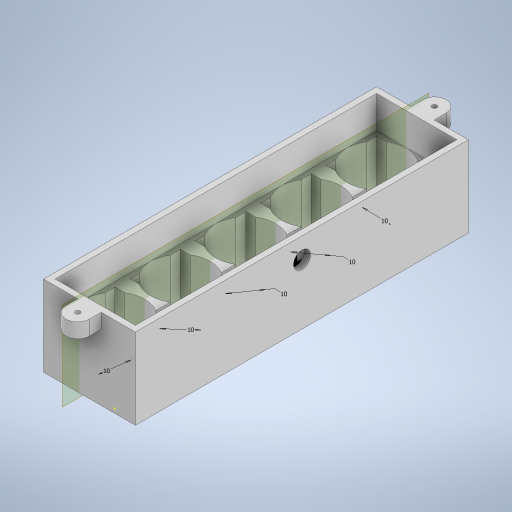
# Autodesk Inventor part: Suporte 4 EletroImã
Saved by Autodesk Inventor 2023 (Build 270158000, 158)
## iProperties
Created: 2023-03-28
Part Number: Suporte 4 EletroImã
Material: Genérico
Document SubType Name: Modeling
Designer: Inteli
Density: 1 g/cm^3
Appearance: Padrão
Author: Inteli
## iProperties of the stored document Suporte 4 EletroImã_3DPrint.ipt
Created: 2023-03-29
Part Number: Suporte 4 EletroImã_3DPrint
Material: Genérico
Document SubType Name: Modeling
Designer: Inteli
Density: 1 g/cm^3
Appearance: Padrão
Author: Inteli
Autodesk Inventor part; units mm, degrees
ref_plane "YZ Plane" through (0, 0, 0) normal (1, 0, 0) x (0, 1, 0)
ref_plane "XZ Plane" through (0, 0, 0) normal (0, 1, 0) x (-1, 0, 0)
ref_plane "XY Plane" through (0, 0, 0) normal (0, 0, 1) x (1, 0, 0)
sketch "Esboço1" plane through (0, 0, 0) normal (0, 1, 0) x (-1, 0, 0)
  circle A0 centre (12.15, -12.15) radius 10.15
  line L0 (0, 0) -> (24.3, 0)
  line L1 (24.3, 0) -> (24.3, -113.5)
  line L2 (24.3, -113.5) -> (0, -113.5)
  line L3 (0, -113.5) -> (0, 0)
  line L4 (20.8, -20.8) -> (3.5, -20.8)
  line L5 (3.5, -20.8) -> (3.5, -3.5)
  line L6 (3.5, -3.5) -> (20.8, -3.5)
  line L7 (20.8, -3.5) -> (20.8, -20.8)
  circle A1 centre (12.15, -34.45) radius 10.15
  line L8 (20.8, -43.1) -> (3.5, -43.1)
  line L9 (3.5, -43.1) -> (3.5, -25.8)
  line L10 (3.5, -25.8) -> (20.8, -25.8)
  line L11 (20.8, -25.8) -> (20.8, -43.1)
  circle A2 centre (12.15, -56.75) radius 10.15
  line L12 (20.8, -65.4) -> (3.5, -65.4)
  line L13 (3.5, -65.4) -> (3.5, -48.1)
  line L14 (3.5, -48.1) -> (20.8, -48.1)
  line L15 (20.8, -48.1) -> (20.8, -65.4)
  circle A3 centre (12.15, -79.05) radius 10.15
  line L16 (20.8, -87.7) -> (3.5, -87.7)
  line L17 (3.5, -87.7) -> (3.5, -70.4)
  line L18 (3.5, -70.4) -> (20.8, -70.4)
  line L19 (20.8, -70.4) -> (20.8, -87.7)
  line L20 (0, -113.5) -> (-7, -113.5)
  line L21 (-7, -113.5) -> (-7, 0)
  line L22 (-7, 0) -> (0, 0)
  line L23 (0, -111.5) -> (-5, -111.5)
  line L24 (-5, -111.5) -> (-5, -2)
  line L25 (-5, -2) -> (0, -2)
  circle A4 centre (12.15, -101.35) radius 10.15
  line L26 (20.8, -110) -> (3.5, -110)
  line L27 (3.5, -110) -> (3.5, -92.7)
  line L28 (3.5, -92.7) -> (20.8, -92.7)
  line L29 (20.8, -92.7) -> (20.8, -110)
  point P0 (20.8, -84.3604)
  point P1 (17.4604, -87.7)
  point P2 (6.8396, -87.7)
  point P3 (3.5, -84.3604)
  point P4 (3.5, -73.7396)
  point P5 (6.8396, -70.4)
  point P6 (17.4604, -70.4)
  point P7 (20.8, -73.7396)
  point P8 (20.8, -62.0604)
  point P9 (17.4604, -65.4)
  point P10 (6.8396, -65.4)
  point P11 (3.5, -62.0604)
  point P12 (3.5, -51.4396)
  point P13 (6.8396, -48.1)
  point P14 (17.4604, -48.1)
  point P15 (20.8, -51.4396)
  point P16 (20.8, -39.7604)
  point P17 (17.4604, -43.1)
  point P18 (6.8396, -43.1)
  point P19 (3.5, -39.7604)
  point P20 (3.5, -29.1396)
  point P21 (6.8396, -25.8)
  point P22 (17.4604, -25.8)
  point P23 (20.8, -29.1396)
  point P24 (20.8, -17.4604)
  point P25 (17.4604, -20.8)
  point P26 (6.8396, -20.8)
  point P27 (3.5, -17.4604)
  point P28 (3.5, -6.8396)
  point P29 (6.8396, -3.5)
  point P30 (17.4604, -3.5)
  point P31 (20.8, -6.8396)
  point P32 (6.8396, -62.0604)
  point P33 (0, -111.5)
  point P34 (6.8396, -110)
  point P35 (3.5, -106.6604)
  point P36 (3.5, -96.0396)
  point P37 (6.8396, -92.7)
  point P38 (17.4604, -92.7)
  point P39 (20.8, -96.0396)
  point P40 (20.8, -106.6604)
  point P41 (17.4604, -110)
  dimension "d0" = 20.3
  dimension "d24" = 22.3
  dimension "d39" = 12.15
  dimension "d41" = 7
  dimension "d42" = 2
  dimension "d96" = 3.5
  dimension "d102" = 5
  constraints: 60 end point, 6 perpendicular, 5 centre point, 5 horizontal, 4 parallel, 1 vertical, 32 other
  measures "d0" diameter of A0
  measures "d24" distance of A0.centre A1.centre
  measures "d39" distance from line of L3 A3.centre
  measures "d41" distance of L2.end L20.end
  measures "d42" distance between parallel lines of L20 L23
  measures "d96" distance between parallel lines of L0 L6
  measures "d102" distance between parallel lines of L28 L16
extrude "Base" add sketch "Esboço1" along normal blind 26 contours L0 L1 L2 L3 | L3 L25 L24 L23 L20 L21 L22
sketch "Esboço2" plane through (0, 0, 0) normal (0, -1, 0) x (1, 0, 0)
  line L0 (-24.3, 0) -> (-24.3, -113.5)
  line L1 (-24.3, -113.5) -> (7, -113.5)
  line L2 (7, 0) -> (7, -113.5) projected
  line L3 (7, 0) -> (7, -113.5)
  line L4 (-24.3, 0) -> (7, 0) projected
  line L5 (7, 0) -> (-24.3, 0)
  constraints: 8 end point, 1 horizontal, 1 point on line, 1 vertical
extrude "Fundo" add sketch "Esboço2" along normal blind 1.5
sketch "Esboço3" plane through (0, 0, 0) normal (0, 1, 0) x (1, 0, 0)
  arc A0 (-6.8396, 20.8) -> (-17.4604, 20.8) centre (-12.15, 12.15) ccw projected
  circle A1 centre (-12.15, 12.15) radius 5
  arc A2 (-6.8396, 43.1) -> (-17.4604, 43.1) centre (-12.15, 34.45) ccw projected
  circle A3 centre (-12.15, 34.45) radius 5
  arc A4 (-6.8396, 65.4) -> (-17.4604, 65.4) centre (-12.15, 56.75) ccw projected
  circle A5 centre (-12.15, 56.75) radius 5
  arc A6 (-6.8396, 87.7) -> (-17.4604, 87.7) centre (-12.15, 79.05) ccw projected
  circle A7 centre (-12.15, 79.05) radius 5
  arc A8 (-20.8, 106.6604) -> (-20.8, 96.0396) centre (-12.15, 101.35) ccw projected
  circle A9 centre (-12.15, 101.35) radius 5
  point P0 (0, 0)
  dimension "d33" = 10
  dimension "d34" = 10
  dimension "d35" = 10
  dimension "d36" = 10
  dimension "d104" = 10
  constraints: 5 centre point, 5 coincident
  measures "d33" diameter of A1
  measures "d34" diameter of A3
  measures "d35" diameter of A5
  measures "d36" diameter of A7
  measures "d104" diameter of A9
extrude "Furo Fundo" cut sketch "Esboço3" against normal up to surface (1.5 mm away)
sketch "Esboço4" plane through (0, 26, 0) normal (0, 1, 0) x (1, 0, 0)
  line L0 (-3.5, 3.5) -> (-6.8396, 3.5) projected
  line L1 (-6.8396, 17.4604) -> (0, 17.4604)
  line L2 (0, 17.4604) -> (0, 29.1396)
  line L3 (0, 29.1396) -> (-6.8396, 29.1396)
  line L4 (-6.8396, 29.1396) -> (-6.8396, 17.4604)
  line L5 (-6.8396, 39.7604) -> (0, 39.7604)
  line L6 (0, 39.7604) -> (0, 51.4396)
  line L7 (0, 51.4396) -> (-6.8396, 51.4396)
  line L8 (-6.8396, 51.4396) -> (-6.8396, 39.7604)
  line L9 (-6.8396, 62.0604) -> (0, 62.0604)
  line L10 (0, 62.0604) -> (0, 73.7396)
  line L11 (0, 73.7396) -> (-6.8396, 73.7396)
  line L12 (-6.8396, 73.7396) -> (-6.8396, 62.0604)
  line L13 (-6.8396, 84.3606) -> (0, 84.3606)
  line L14 (0, 84.3606) -> (0, 96.0399)
  line L15 (0, 96.0399) -> (-6.8396, 96.0399)
  line L16 (-6.8396, 96.0399) -> (-6.8396, 84.3606)
  point P0 (0, 0)
  point P1 (-6.8396, 87.7)
  point P2 (-3.5, 17.4604)
  point P3 (-6.8396, 29.1396)
  point P4 (-6.8396, 51.4396)
  point P5 (-6.8396, 73.7396)
  constraints: 32 end point, 8 parallel, 4 horizontal, 4 perpendicular, 1 point on line
extrude "Espaço Fio E.I" cut sketch "Esboço4" against normal blind 14
sketch "Esboço5" plane through (0, 26, 0) normal (0, 1, 0) x (1, 0, 0)
  arc A0 (-17.4604, 3.5) -> (-6.8396, 3.5) centre (-12.15, 12.15) ccw projected
  arc A1 (-6.8396, 87.7) -> (-17.4604, 87.7) centre (-12.15, 79.05) ccw projected
  arc A2 (-20.8, 84.3604) -> (-20.8, 73.7396) centre (-12.15, 79.05) ccw projected
  line L0 (5, 2) -> (-22.3, 2)
  line L1 (-22.3, 2) -> (-22.3, 111.5)
  line L2 (-22.3, 111.5) -> (5, 111.5)
  line L3 (5, 111.5) -> (5, 2)
  line L4 (5, 111.5) -> (5, 2) projected
  line L5 (0, 111.5) -> (5, 111.5) projected
  point P0 (0, 0)
  constraints: 8 end point, 2 parallel, 1 horizontal, 1 perpendicular
extrude "Suporte PCB" cut sketch "Esboço5" against normal blind 11
sketch "Esboço6" plane through (5, 26, -111.5) normal (-1, 0, 0) x (0, 0, 1)
  circle A0 centre (54.75, -7) radius 2.85
  line L0 (77.05, -11) -> (54.75, -11) projected
  line L1 (-2, 0) -> (111.5, 0) projected
  point P0 (111.5, -26)
  dimension "d49" = 5.7
  constraints: 1 centre point
  measures "d49" diameter of A0
extrude "Furo LED" cut sketch "Esboço6" against normal up to surface (2 mm away)
sketch "Esboço7" plane through (0, 26, 0) normal (0, 1, 0) x (1, 0, 0)
  line L0 (-22.3, 2) -> (-22.3, 111.5) projected
  line L1 (5, 111.5) -> (5, 2) projected
  line L2 (-24.3, 0) -> (-24.3, 113.5) projected
  line L3 (-8.65, 0) -> (-12.65, 0)
  line L4 (-12.65, 0) -> (-12.65, -4)
  line L5 (-8.65, -8) -> (-8.65, -8)
  line L6 (-4.65, -4) -> (-4.65, 0)
  line L7 (-4.65, 0) -> (-8.65, 0)
  circle A0 centre (-8.65, -4) radius 0.8
  arc A1 (-8.65, -8) -> (-4.65, -4) centre (-8.65, -4) ccw
  arc A2 (-12.65, -4) -> (-8.65, -8) centre (-8.65, -4) ccw
  circle A3 centre (-12.15, 56.75) radius 5 projected
  line L8 (-12.15, 56.75) -> (-4.65, 56.75)
  line L9 (-12.65, 113.5) -> (-12.65, 117.5)
  line L10 (-8.65, 113.5) -> (-12.65, 113.5)
  line L11 (-4.65, 117.5) -> (-4.65, 113.5)
  line L12 (-4.65, 113.5) -> (-8.65, 113.5)
  circle A4 centre (-8.65, 117.5) radius 0.8
  arc A5 (-4.65, 117.5) -> (-8.65, 121.5) centre (-8.65, 117.5) ccw
  arc A6 (-8.65, 121.5) -> (-12.65, 117.5) centre (-8.65, 117.5) ccw
  line L13 (-8.65, 121.5) -> (-8.65, 121.5)
  point P0 (-12.65, -8)
  point P1 (-4.65, -8)
  point P2 (-4.65, 121.5)
  point P3 (-12.65, 121.5)
  constraints: 22 end point, 12 symmetric about line, 8 point on circle, 8 point on line, 6 centre point, 1 horizontal, 3 other
extrude "Suporte Parafuso" add sketch "Esboço7" against normal blind 5 contours L7 L6 A1 A2 L4 L3 | L9 A6 A5 L11 L12 L10
ref_plane "Plano de trabalho1" through (-12.15, 26, -113.5) normal (-1, 0, 0) x (0, 0, 1)
sketch "Esboço8" plane through (-12.15, 26, -113.5) normal (-1, 0, 0) x (0, 0, 1)
  line L0 (5.8639, -26.5) -> (3.2916, -27.5)
  line L1 (113.5, -27.5) -> (0, -27.5) projected
  line L2 (3.2916, -27.5) -> (7.15, -27.5)
  line L3 (111.5, -26) -> (2, -26) projected
  line L4 (12.15, -26.5) -> (12.15, -27.5)
  line L5 (12.15, -27.5) -> (3.2916, -27.5)
  line L6 (29.45, -26) -> (39.45, -26) projected
  line L7 (29.45, -26) -> (34.45, -26)
  line L8 (12.15, -26.5) -> (5.8639, -26.5)
  line L9 (51.75, -26) -> (61.75, -26) projected
  line L10 (51.75, -26) -> (56.75, -26)
  line L11 (13.8435, -26.5) -> (16.8286, -26.5)
  line L12 (16.8286, -26.5) -> (110.2631, -26.5)
  line L13 (110.2631, -26.5) -> (16.3892, -26.5)
  line L14 (84.05, -27.5) -> (74.05, -27.5) projected
  line L15 (34.45, -26.5) -> (34.45, -27.5)
  line L16 (28.1639, -26.5) -> (25.5916, -27.5)
  line L17 (25.5916, -27.5) -> (29.45, -27.5)
  line L18 (34.45, -27.5) -> (25.5916, -27.5)
  line L19 (34.45, -26.5) -> (28.1639, -26.5)
  line L20 (56.75, -26.5) -> (56.75, -27.5)
  line L21 (50.4639, -26.5) -> (47.8916, -27.5)
  line L22 (47.8916, -27.5) -> (51.75, -27.5)
  line L23 (56.75, -27.5) -> (47.8916, -27.5)
  line L24 (56.75, -26.5) -> (50.4639, -26.5)
  line L25 (79.05, -26.5) -> (79.05, -27.5)
  line L26 (72.7639, -26.5) -> (70.1916, -27.5)
  line L27 (70.1916, -27.5) -> (74.05, -27.5)
  line L28 (79.05, -27.5) -> (70.1916, -27.5)
  line L29 (79.05, -26.5) -> (72.7639, -26.5)
  line L30 (101.35, -26.5) -> (101.35, -27.5)
  line L31 (95.0639, -26.5) -> (92.4916, -27.5)
  line L32 (92.4916, -27.5) -> (96.35, -27.5)
  line L33 (101.35, -27.5) -> (92.4916, -27.5)
  line L34 (101.35, -26.5) -> (95.0639, -26.5)
  point P0 (113.5, -26)
  point P1 (17.15, -26)
  point P2 (17.15, -26)
  point P3 (79.05, -27.5)
  point P4 (101.3467, -26)
  point P5 (79.05, -26)
  point P6 (25.5916, -27.5)
  point P7 (34.45, -27.5)
  point P8 (34.45, -26.5)
  dimension "d117" = 22.3
  constraints: 60 end point, 5 coincident, 4 point on line, 3 horizontal, 3 midpoint, 2 perpendicular, 1 parallel, 43 other
  measures "d117" distance of L0.end L16.end
revolve "Revolução2" cut sketch "Esboço8" angle 360 about axis through (-12.15, -0.5, -101.35) along (0, -1, 0) contours L8 L4 L1 L0
revolve "Revolução3" cut sketch "Esboço8" angle 360 about axis through (-12.15, -0.5, -79.05) along (0, -1, 0) contours L16 L12 L15 L1
revolve "Revolução4" cut sketch "Esboço8" angle 360 about axis through (-12.15, -0.5, -56.75) along (0, -1, 0) contours L21 L12 L20 L1
revolve "Revolução5" cut sketch "Esboço8" angle 360 about axis through (-12.15, -0.5, -12.15) along (0, -1, 0) contours L12 L30 L1 L31
revolve "Revolução6" cut sketch "Esboço8" angle 360 about axis through (-12.15, -0.5, -34.45) along (0, -1, 0) contours L12 L25 L1 L26
